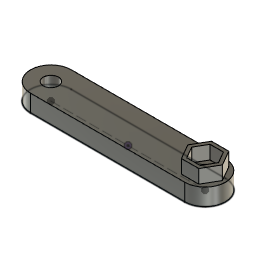
Camera Stand Part 3 (Autodesk Fusion 360 design; units mm, degrees)
Autodesk Fusion 360 part; units mm, degrees
note: some values were not read from the file. Set by a fixed rule: the direction of a hole.
sketch "Sketch1" plane through (0, 0, 0) normal (0, 0, 1) x (1, 0, 0)
  line L0 (-22.75, -6) -> (22.75, -6)
  arc A0 (22.75, -6) -> (22.75, 6) centre (22.75, 0) ccw
  line L1 (22.75, 6) -> (-22.75, 6)
  arc A1 (-22.75, 6) -> (-22.75, -6) centre (-22.75, 0) ccw
  line L2 (-22.75, 0) -> (22.75, 0) construction
  dimension "d1" = 45.5
  dimension "d2" = 12
  constraint tangent L0 A0
  constraint tangent A0 L1
  constraint parallel L0 L1
  constraint tangent L1 A1
  constraint tangent L0 A1
  constraint horizontal L2
  constraint midpoint L2 origin
  measures "d1" distance of A1.centre A0.centre
  measures "d2" distance of L0 L1
extrude "Extrude1" add sketch "Sketch1" along normal blind 5
hole "Hole1" at (22.75, 0, 0) at (-22.75, 0, 0) direction (0, 0, 1) diameter 4.5 depth 8 tip angle 118
sketch "Sketch4" plane through (0, 0, 5) normal (0, 0, 1) x (-1, 0, 0)
  circle A0 centre (-22.75, 0) radius 2.25
  circle A1 centre (22.75, 0) radius 2.25
  arc A2 (22.75, -6) -> (22.75, 6) centre (22.75, 0) ccw
  line L0 (22.75, 6) -> (-22.75, 6)
  arc A3 (-22.75, 6) -> (-22.75, -6) centre (-22.75, 0) ccw
  line L1 (-22.75, -6) -> (22.75, -6)
  line L2 (-26.7048, 0) -> (-24.7274, -3.425)
  line L3 (-24.7274, -3.425) -> (-20.7726, -3.425)
  line L4 (-20.7726, -3.425) -> (-18.7952, 0)
  line L5 (-18.7952, 0) -> (-20.7726, 3.425)
  line L6 (-20.7726, 3.425) -> (-24.7274, 3.425)
  line L7 (-24.7274, 3.425) -> (-26.7048, 0)
  line L8 (-20.1952, 4.425) -> (-25.3048, 4.425)
  line L9 (-25.3048, 4.425) -> (-27.8595, 0)
  line L10 (-27.8595, 0) -> (-25.3048, -4.425)
  line L11 (-25.3048, -4.425) -> (-20.1952, -4.425)
  line L12 (-20.1952, -4.425) -> (-17.6405, 0)
  line L13 (-17.6405, 0) -> (-20.1952, 4.425)
  point P0 (-22.75, 0)
  dimension "d8" = 6.85
  dimension "d9" = 1
  constraint coincident P0 A0.centre
  measures "d8" distance of L3 L6
extrude "Extrude2" add sketch "Sketch4" along normal blind 4 contours L8 L9 L10 L11 L12 L13
